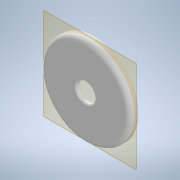
# Autodesk Inventor part: dekieltop
Saved by Autodesk Inventor 2021 (Build 250183000, 183)
## iProperties
Created: 2021-05-20
Part Number: dekieltop
Material: Ogólny
Document SubType Name: Modeling
Designer: Wojciech Wołczek
Density: 1 g/cm^3
Appearance: Domyślna
Author: Wojciech Wołczek
Autodesk Inventor part; units mm, degrees
ref_plane "YZ Plane" through (0, 0, 0) normal (1, 0, 0) x (0, 1, 0)
ref_plane "XZ Plane" through (0, 0, 0) normal (0, 1, 0) x (-1, 0, 0)
ref_plane "XY Plane" through (0, 0, 0) normal (0, 0, 1) x (1, 0, 0)
sketch "Szkic1" plane through (0, 0, 0) normal (0, 0, 1) x (1, 0, 0)
  circle A0 centre (0, 0) radius 90 projected
  circle A1 centre (0, 0) radius 90
  circle A2 centre (0, 0) radius 95
  point P0 (0, 0)
  dimension "d0" = 190
  constraints: 2 centre point, 2 coincident, 1 concentric
  measures "d0" diameter of A2
extrude "Wyciągnięcie proste1" add sketch "Szkic1" against normal blind 10
ref_plane "Płaszczyzna konstrukcyjna1" through (0, 0, 0) normal (0, 0, 1) x (1, 0, 0)
sketch "Szkic2" plane through (0, 0, 0) normal (0, 0, 1) x (1, 0, 0)
  circle A0 centre (0, 0) radius 95
  circle A1 centre (0, 0) radius 20
  dimension "d3" = 40
  constraints: 2 centre point, 2 coincident
  measures "d3" diameter of A1
extrude "Wyciągnięcie proste2" add sketch "Szkic2" along normal blind 10
fillet "Zaokrąglenie1" radius 10 1 edges at (-95, 0, 10)
chamfer "Faza1" distance 2 angle 45 1 edges at (-95, 0, -10)
chamfer "Faza2" distance 2 angle 45 2 edges at (-20, 0, 0) (-20, 0, 10)
